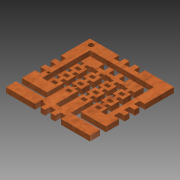
# Autodesk Inventor part: mech
Saved by Autodesk Inventor 2014 SP1 (Build 180222100, 222)
## iProperties
Created: 2015-02-17
Part Number: mech
Material: Wood (Cherry)
Document SubType Name: Modeling
Designer: Erin
Density: 0.63 g/cm^3
Appearance: Cherry - Natural Low Gloss
Author: Erin
Autodesk Inventor part; units mm, degrees
ref_plane "YZ Plane" through (0, 0, 0) normal (1, 0, 0) x (0, 1, 0)
ref_plane "XZ Plane" through (0, 0, 0) normal (0, 1, 0) x (-1, 0, 0)
ref_plane "XY Plane" through (0, 0, 0) normal (0, 0, 1) x (1, 0, 0)
sketch "slots" plane through (0, 0, 0) normal (0, 0, 1) x (1, 0, 0)
  line L0 (61.2817, 31.2571) -> (64.5817, 31.2571)
  line L1 (64.5817, 31.2571) -> (64.5817, 28.1071)
  line L2 (64.5817, 28.1071) -> (61.2817, 28.1071)
  line L3 (61.2817, 28.1071) -> (61.2817, 31.2571)
  line L4 (68.9317, 33.8834) -> (68.9317, 26.9198) construction
  line L5 (67.2817, 31.2571) -> (70.5817, 31.2571)
  line L6 (70.5817, 31.2571) -> (70.5817, 28.1071)
  line L7 (70.5817, 28.1071) -> (67.2817, 28.1071)
  line L8 (67.2817, 28.1071) -> (67.2817, 31.2571)
  line L9 (73.2817, 31.2571) -> (76.5817, 31.2571)
  line L10 (76.5817, 31.2571) -> (76.5817, 28.1071)
  line L11 (76.5817, 28.1071) -> (73.2817, 28.1071)
  line L12 (73.2817, 28.1071) -> (73.2817, 31.2571)
  line L13 (68.9317, 28.1071) -> (68.9317, 27.1937) construction
  point P0 (68.8645, 30.3856)
  dimension "d2" = 3.3
  dimension "d3" = 3.15
  dimension "d99" = 2.7
  dimension "d100" = 2.7
  measures "d2" distance of L1.end L2.end
  measures "d3" distance of L0.end L1.end
  measures "d99" distance between parallel lines of L8 L1
  measures "d100" distance between parallel lines of L12 L6
sketch "flexure" plane through (0, 0, 0) normal (0, 0, 1) x (1, 0, 0)
  line L0 (49.9032, 40.0133) -> (55.9032, 40.0133)
  line L1 (55.9032, 40.0133) -> (55.9032, 19.5133)
  line L2 (55.9032, 19.5133) -> (49.9032, 19.5133)
  line L3 (49.9032, 19.5133) -> (49.9032, 40.0133)
  line L4 (49.9032, 32.5133) -> (52.085, 32.5133)
  line L5 (52.085, 32.5133) -> (52.085, 30.5133)
  line L6 (52.085, 30.5133) -> (49.9032, 30.5133)
  line L7 (49.9032, 30.5133) -> (49.9032, 32.5133)
  line L8 (53.7214, 30.5133) -> (53.7214, 32.5133)
  line L9 (55.9032, 30.5133) -> (53.7214, 30.5133)
  line L10 (53.7214, 32.5133) -> (55.9032, 32.5133)
  line L11 (55.9032, 32.5133) -> (55.9032, 30.5133)
  line L12 (51.5395, 29.0133) -> (54.2668, 29.0133)
  line L13 (54.2668, 29.0133) -> (54.2668, 27.0133)
  line L14 (54.2668, 27.0133) -> (51.5395, 27.0133)
  line L15 (51.5395, 27.0133) -> (51.5395, 29.0133)
  line L16 (49.9032, 29.7633) -> (55.9032, 29.7633) construction
  line L17 (55.9032, 29.7633) -> (49.9032, 29.7633) construction
  line L18 (53.7214, 25.5133) -> (55.9032, 25.5133)
  line L19 (55.9032, 25.5133) -> (55.9032, 23.5133)
  line L20 (55.9032, 23.5133) -> (53.7214, 23.5133)
  line L21 (53.7214, 23.5133) -> (53.7214, 25.5133)
  line L22 (51.5395, 22.0133) -> (54.2668, 22.0133)
  line L23 (54.2668, 22.0133) -> (54.2668, 20.0133)
  line L24 (54.2668, 20.0133) -> (51.5395, 20.0133)
  line L25 (51.5395, 20.0133) -> (51.5395, 22.0133)
  line L26 (49.9032, 25.5133) -> (52.085, 25.5133)
  line L27 (52.085, 25.5133) -> (52.085, 23.5133)
  line L28 (52.085, 23.5133) -> (49.9032, 23.5133)
  line L29 (49.9032, 23.5133) -> (49.9032, 25.5133)
  line L30 (49.9032, 22.7633) -> (55.9032, 22.7633) construction
  line L31 (55.9032, 22.7633) -> (49.9032, 22.7633) construction
  line L32 (53.7214, 39.5133) -> (55.9032, 39.5133)
  line L33 (55.9032, 39.5133) -> (55.9032, 37.5133)
  line L34 (55.9032, 37.5133) -> (53.7214, 37.5133)
  line L35 (53.7214, 37.5133) -> (53.7214, 39.5133)
  line L36 (51.5395, 36.0133) -> (54.2668, 36.0133)
  line L37 (54.2668, 36.0133) -> (54.2668, 34.0133)
  line L38 (54.2668, 34.0133) -> (51.5395, 34.0133)
  line L39 (51.5395, 34.0133) -> (51.5395, 36.0133)
  line L40 (49.9032, 39.5133) -> (52.085, 39.5133)
  line L41 (52.085, 39.5133) -> (52.085, 37.5133)
  line L42 (52.085, 37.5133) -> (49.9032, 37.5133)
  line L43 (49.9032, 37.5133) -> (49.9032, 39.5133)
  line L44 (49.9032, 36.7633) -> (55.9032, 36.7633) construction
  line L45 (55.9032, 36.7633) -> (49.9032, 36.7633) construction
  line L46 (53.7214, 32.5133) -> (55.9032, 32.5133)
  line L47 (55.9032, 32.5133) -> (55.9032, 30.5133)
  line L48 (55.9032, 30.5133) -> (53.7214, 30.5133)
  line L49 (53.7214, 30.5133) -> (53.7214, 32.5133)
  line L50 (51.5395, 29.0133) -> (54.2668, 29.0133)
  line L51 (54.2668, 29.0133) -> (54.2668, 27.0133)
  line L52 (54.2668, 27.0133) -> (51.5395, 27.0133)
  line L53 (51.5395, 27.0133) -> (51.5395, 29.0133)
  line L54 (49.9032, 32.5133) -> (52.085, 32.5133)
  line L55 (52.085, 32.5133) -> (52.085, 30.5133)
  line L56 (52.085, 30.5133) -> (49.9032, 30.5133)
  line L57 (49.9032, 30.5133) -> (49.9032, 32.5133)
  line L58 (49.9032, 29.7633) -> (55.9032, 29.7633) construction
  line L59 (55.9032, 29.7633) -> (49.9032, 29.7633) construction
  point P0 (52.8239, 25.8216)
  dimension "d22" = 6
  dimension "d24" = 2.1818
  dimension "d27" = 3.8182
  dimension "d32" = 1.6364
  dimension "d33" = 2.7273
  dimension "d41" = 2
  dimension "d42" = 2
  dimension "d43" = 1.5
  dimension "d93" = 20.5
  dimension "d106" = 7
  dimension "d109" = 7
  dimension "d117" = 11
  measures "d22" distance of L1.end L2.end
  measures "d24" distance of L4.start L4.end
  measures "d27" distance of L6.end L9.end
  measures "d32" distance between parallel lines of L15 L3
  measures "d33" distance of L12.start L12.end
  measures "d41" distance of L4.end L5.end
  measures "d42" distance of L12.end L13.end
  measures "d43" distance between parallel lines of L12 L6
  measures "d93" distance of L0.end L1.end
  measures "d106" distance of L10.start L18.start
  measures "d109" distance of L10.start L32.start
  measures "d117" distance between parallel lines of L12 L0
sketch "Sketch1" plane through (0, 0, 0) normal (0, 0, 1) x (1, 0, 0)
  line L0 (-25, 25) -> (25, 25) construction
  line L1 (25, 25) -> (25, -25) construction
  line L2 (25, -25) -> (-25, -25) construction
  line L3 (-25, -25) -> (-25, 25) construction
  line L4 (-25, -25) -> (25, -25)
  line L5 (25, -25) -> (25, -19)
  line L6 (25, -19) -> (-25, -19)
  line L7 (-25, -19) -> (-25, -25)
  line L8 (0, 33.5916) -> (0, -39.9789) construction
  line L9 (-35.9054, 0) -> (42.6007, 0) construction
  line L10 (-25, 25) -> (25, 25)
  line L11 (25, 25) -> (25, 19)
  line L12 (25, 19) -> (-25, 19)
  line L13 (-25, 19) -> (-25, 25)
  line L14 (-25, 19) -> (-19, 19)
  line L15 (-19, 19) -> (-19, -15.5)
  line L16 (-19, -15.5) -> (-25, -15.5)
  line L17 (-25, -15.5) -> (-25, 19)
  line L18 (-19, -15.5) -> (-10, -15.5)
  line L19 (-10, -15.5) -> (-10, -9.5)
  line L20 (-10, -9.5) -> (-19, -9.5)
  line L21 (-19, -9.5) -> (-19, -15.5)
  line L22 (25, 19) -> (19, 19)
  line L23 (19, 19) -> (19, -15.5)
  line L24 (19, -15.5) -> (25, -15.5)
  line L25 (25, -15.5) -> (25, 19)
  line L26 (19, -15.5) -> (10, -15.5)
  line L27 (10, -15.5) -> (10, -9.5)
  line L28 (10, -9.5) -> (19, -9.5)
  line L29 (19, -9.5) -> (19, -15.5)
  line L30 (-16, 16) -> (16, 16)
  line L31 (16, 16) -> (16, 11)
  line L32 (16, 11) -> (-16, 11)
  line L33 (-16, 11) -> (-16, 16)
  line L34 (-7.5, -9.5) -> (-1.5, -9.5)
  line L35 (-1.5, -9.5) -> (-1.5, -19)
  line L36 (-1.5, -19) -> (-7.5, -19)
  line L37 (-7.5, -19) -> (-7.5, -9.5)
  line L38 (1.5, -9.5) -> (7.5, -9.5)
  line L39 (7.5, -9.5) -> (7.5, -19)
  line L40 (7.5, -19) -> (1.5, -19)
  line L41 (1.5, -19) -> (1.5, -9.5)
  line L42 (-68.1542, 16.5688) -> (-29.44, 16.5688) construction
  line L43 (-29.44, 16.5688) -> (-29.44, -5.0786) construction
  line L44 (-29.44, -5.0786) -> (-68.1542, -5.0786) construction
  line L45 (-68.1542, -5.0786) -> (-68.1542, 16.5688) construction
  circle A0 centre (-21.2866, 22) radius 1.5
  line L46 (-7.65, 25) -> (-4.35, 25)
  line L47 (-4.35, 25) -> (-4.35, 21.85)
  line L48 (-4.35, 21.85) -> (-7.65, 21.85)
  line L49 (-7.65, 21.85) -> (-7.65, 25)
  line L50 (0, 27.6263) -> (0, 20.6627) construction
  line L51 (-1.65, 25) -> (1.65, 25)
  line L52 (1.65, 25) -> (1.65, 21.85)
  line L53 (1.65, 21.85) -> (-1.65, 21.85)
  line L54 (-1.65, 21.85) -> (-1.65, 25)
  line L55 (4.35, 25) -> (7.65, 25)
  line L56 (7.65, 25) -> (7.65, 21.85)
  line L57 (7.65, 21.85) -> (4.35, 21.85)
  line L58 (4.35, 21.85) -> (4.35, 25)
  line L59 (0, 21.85) -> (0, 20.9366) construction
  line L60 (-7.65, -21.85) -> (-4.35, -21.85)
  line L61 (-4.35, -21.85) -> (-4.35, -25)
  line L62 (-4.35, -25) -> (-7.65, -25)
  line L63 (-7.65, -25) -> (-7.65, -21.85)
  line L64 (0, -19.2237) -> (0, -26.1873) construction
  line L65 (-1.65, -21.85) -> (1.65, -21.85)
  line L66 (1.65, -21.85) -> (1.65, -25)
  line L67 (1.65, -25) -> (-1.65, -25)
  line L68 (-1.65, -25) -> (-1.65, -21.85)
  line L69 (4.35, -21.85) -> (7.65, -21.85)
  line L70 (7.65, -21.85) -> (7.65, -25)
  line L71 (7.65, -25) -> (4.35, -25)
  line L72 (4.35, -25) -> (4.35, -21.85)
  line L73 (0, -25) -> (0, -25.9134) construction
  line L74 (-25, -7.65) -> (-25, -4.35)
  line L75 (-25, -4.35) -> (-21.85, -4.35)
  line L76 (-21.85, -4.35) -> (-21.85, -7.65)
  line L77 (-21.85, -7.65) -> (-25, -7.65)
  line L78 (-27.6263, 0) -> (-20.6627, 0) construction
  line L79 (-25, -1.65) -> (-25, 1.65)
  line L80 (-25, 1.65) -> (-21.85, 1.65)
  line L81 (-21.85, 1.65) -> (-21.85, -1.65)
  line L82 (-21.85, -1.65) -> (-25, -1.65)
  line L83 (-25, 4.35) -> (-25, 7.65)
  line L84 (-25, 7.65) -> (-21.85, 7.65)
  line L85 (-21.85, 7.65) -> (-21.85, 4.35)
  line L86 (-21.85, 4.35) -> (-25, 4.35)
  line L87 (-21.85, 0) -> (-20.9366, 0) construction
  line L88 (21.85, -7.65) -> (21.85, -4.35)
  line L89 (21.85, -4.35) -> (25, -4.35)
  line L90 (25, -4.35) -> (25, -7.65)
  line L91 (25, -7.65) -> (21.85, -7.65)
  line L92 (19.2237, 0) -> (26.1873, 0) construction
  line L93 (21.85, -1.65) -> (21.85, 1.65)
  line L94 (21.85, 1.65) -> (25, 1.65)
  line L95 (25, 1.65) -> (25, -1.65)
  line L96 (25, -1.65) -> (21.85, -1.65)
  line L97 (21.85, 4.35) -> (21.85, 7.65)
  line L98 (21.85, 7.65) -> (25, 7.65)
  line L99 (25, 7.65) -> (25, 4.35)
  line L100 (25, 4.35) -> (21.85, 4.35)
  line L101 (25, 0) -> (25.9134, 0) construction
  line L102 (-16, 11) -> (-10, 11)
  line L103 (-10, 11) -> (-10, -9.5)
  line L104 (-10, -9.5) -> (-16, -9.5)
  line L105 (-16, -9.5) -> (-16, 11)
  line L106 (-16, 3.5) -> (-13.8182, 3.5)
  line L107 (-13.8182, 3.5) -> (-13.8182, 1.5)
  line L108 (-13.8182, 1.5) -> (-16, 1.5)
  line L109 (-16, 1.5) -> (-16, 3.5)
  line L110 (-12.1818, 1.5) -> (-12.1818, 3.5)
  line L111 (-10, 1.5) -> (-12.1818, 1.5)
  line L112 (-12.1818, 3.5) -> (-10, 3.5)
  line L113 (-10, 3.5) -> (-10, 1.5)
  line L114 (-14.3636, 0) -> (-11.6364, 0)
  line L115 (-11.6364, 0) -> (-11.6364, -2)
  line L116 (-11.6364, -2) -> (-14.3636, -2)
  line L117 (-14.3636, -2) -> (-14.3636, 0)
  line L118 (-16, 0.75) -> (-10, 0.75) construction
  line L119 (-10, 0.75) -> (-16, 0.75) construction
  line L120 (-12.1818, -3.5) -> (-10, -3.5)
  line L121 (-10, -3.5) -> (-10, -5.5)
  line L122 (-10, -5.5) -> (-12.1818, -5.5)
  line L123 (-12.1818, -5.5) -> (-12.1818, -3.5)
  line L124 (-14.3636, -7) -> (-11.6364, -7)
  line L125 (-11.6364, -7) -> (-11.6364, -9)
  line L126 (-11.6364, -9) -> (-14.3636, -9)
  line L127 (-14.3636, -9) -> (-14.3636, -7)
  line L128 (-16, -3.5) -> (-13.8182, -3.5)
  line L129 (-13.8182, -3.5) -> (-13.8182, -5.5)
  line L130 (-13.8182, -5.5) -> (-16, -5.5)
  line L131 (-16, -5.5) -> (-16, -3.5)
  line L132 (-16, -6.25) -> (-10, -6.25) construction
  line L133 (-10, -6.25) -> (-16, -6.25) construction
  line L134 (-12.1818, 10.5) -> (-10, 10.5)
  line L135 (-10, 10.5) -> (-10, 8.5)
  line L136 (-10, 8.5) -> (-12.1818, 8.5)
  line L137 (-12.1818, 8.5) -> (-12.1818, 10.5)
  line L138 (-14.3636, 7) -> (-11.6364, 7)
  line L139 (-11.6364, 7) -> (-11.6364, 5)
  line L140 (-11.6364, 5) -> (-14.3636, 5)
  line L141 (-14.3636, 5) -> (-14.3636, 7)
  line L142 (-16, 10.5) -> (-13.8182, 10.5)
  line L143 (-13.8182, 10.5) -> (-13.8182, 8.5)
  line L144 (-13.8182, 8.5) -> (-16, 8.5)
  line L145 (-16, 8.5) -> (-16, 10.5)
  line L146 (-16, 7.75) -> (-10, 7.75) construction
  line L147 (-10, 7.75) -> (-16, 7.75) construction
  line L148 (-12.1818, 3.5) -> (-10, 3.5)
  line L149 (-10, 3.5) -> (-10, 1.5)
  line L150 (-10, 1.5) -> (-12.1818, 1.5)
  line L151 (-12.1818, 1.5) -> (-12.1818, 3.5)
  line L152 (-14.3636, 0) -> (-11.6364, 0)
  line L153 (-11.6364, 0) -> (-11.6364, -2)
  line L154 (-11.6364, -2) -> (-14.3636, -2)
  line L155 (-14.3636, -2) -> (-14.3636, 0)
  line L156 (-16, 3.5) -> (-13.8182, 3.5)
  line L157 (-13.8182, 3.5) -> (-13.8182, 1.5)
  line L158 (-13.8182, 1.5) -> (-16, 1.5)
  line L159 (-16, 1.5) -> (-16, 3.5)
  line L160 (-16, 0.75) -> (-10, 0.75) construction
  line L161 (-10, 0.75) -> (-16, 0.75) construction
  line L162 (10, 11) -> (16, 11)
  line L163 (16, 11) -> (16, -9.5)
  line L164 (16, -9.5) -> (10, -9.5)
  line L165 (10, -9.5) -> (10, 11)
  line L166 (10, 3.5) -> (12.1818, 3.5)
  line L167 (12.1818, 3.5) -> (12.1818, 1.5)
  line L168 (12.1818, 1.5) -> (10, 1.5)
  line L169 (10, 1.5) -> (10, 3.5)
  line L170 (13.8182, 1.5) -> (13.8182, 3.5)
  line L171 (16, 1.5) -> (13.8182, 1.5)
  line L172 (13.8182, 3.5) -> (16, 3.5)
  line L173 (16, 3.5) -> (16, 1.5)
  line L174 (11.6364, 0) -> (14.3636, 0)
  line L175 (14.3636, 0) -> (14.3636, -2)
  line L176 (14.3636, -2) -> (11.6364, -2)
  line L177 (11.6364, -2) -> (11.6364, 0)
  line L178 (10, 0.75) -> (16, 0.75) construction
  line L179 (16, 0.75) -> (10, 0.75) construction
  line L180 (13.8182, -3.5) -> (16, -3.5)
  line L181 (16, -3.5) -> (16, -5.5)
  line L182 (16, -5.5) -> (13.8182, -5.5)
  line L183 (13.8182, -5.5) -> (13.8182, -3.5)
  line L184 (11.6364, -7) -> (14.3636, -7)
  line L185 (14.3636, -7) -> (14.3636, -9)
  line L186 (14.3636, -9) -> (11.6364, -9)
  line L187 (11.6364, -9) -> (11.6364, -7)
  line L188 (10, -3.5) -> (12.1818, -3.5)
  line L189 (12.1818, -3.5) -> (12.1818, -5.5)
  line L190 (12.1818, -5.5) -> (10, -5.5)
  line L191 (10, -5.5) -> (10, -3.5)
  line L192 (10, -6.25) -> (16, -6.25) construction
  line L193 (16, -6.25) -> (10, -6.25) construction
  line L194 (13.8182, 10.5) -> (16, 10.5)
  line L195 (16, 10.5) -> (16, 8.5)
  line L196 (16, 8.5) -> (13.8182, 8.5)
  line L197 (13.8182, 8.5) -> (13.8182, 10.5)
  line L198 (11.6364, 7) -> (14.3636, 7)
  line L199 (14.3636, 7) -> (14.3636, 5)
  line L200 (14.3636, 5) -> (11.6364, 5)
  line L201 (11.6364, 5) -> (11.6364, 7)
  line L202 (10, 10.5) -> (12.1818, 10.5)
  line L203 (12.1818, 10.5) -> (12.1818, 8.5)
  line L204 (12.1818, 8.5) -> (10, 8.5)
  line L205 (10, 8.5) -> (10, 10.5)
  line L206 (10, 7.75) -> (16, 7.75) construction
  line L207 (16, 7.75) -> (10, 7.75) construction
  line L208 (13.8182, 3.5) -> (16, 3.5)
  line L209 (16, 3.5) -> (16, 1.5)
  line L210 (16, 1.5) -> (13.8182, 1.5)
  line L211 (13.8182, 1.5) -> (13.8182, 3.5)
  line L212 (11.6364, 0) -> (14.3636, 0)
  line L213 (14.3636, 0) -> (14.3636, -2)
  line L214 (14.3636, -2) -> (11.6364, -2)
  line L215 (11.6364, -2) -> (11.6364, 0)
  line L216 (10, 3.5) -> (12.1818, 3.5)
  line L217 (12.1818, 3.5) -> (12.1818, 1.5)
  line L218 (12.1818, 1.5) -> (10, 1.5)
  line L219 (10, 1.5) -> (10, 3.5)
  line L220 (10, 0.75) -> (16, 0.75) construction
  line L221 (16, 0.75) -> (10, 0.75) construction
  line L222 (1.5, 11) -> (7.5, 11)
  line L223 (7.5, 11) -> (7.5, -9.5)
  line L224 (7.5, -9.5) -> (1.5, -9.5)
  line L225 (1.5, -9.5) -> (1.5, 11)
  line L226 (1.5, 3.5) -> (3.6818, 3.5)
  line L227 (3.6818, 3.5) -> (3.6818, 1.5)
  line L228 (3.6818, 1.5) -> (1.5, 1.5)
  line L229 (1.5, 1.5) -> (1.5, 3.5)
  line L230 (5.3182, 1.5) -> (5.3182, 3.5)
  line L231 (7.5, 1.5) -> (5.3182, 1.5)
  line L232 (5.3182, 3.5) -> (7.5, 3.5)
  line L233 (7.5, 3.5) -> (7.5, 1.5)
  line L234 (3.1364, 0) -> (5.8636, 0)
  line L235 (5.8636, 0) -> (5.8636, -2)
  line L236 (5.8636, -2) -> (3.1364, -2)
  line L237 (3.1364, -2) -> (3.1364, 0)
  line L238 (1.5, 0.75) -> (7.5, 0.75) construction
  line L239 (7.5, 0.75) -> (1.5, 0.75) construction
  line L240 (5.3182, -3.5) -> (7.5, -3.5)
  line L241 (7.5, -3.5) -> (7.5, -5.5)
  line L242 (7.5, -5.5) -> (5.3182, -5.5)
  line L243 (5.3182, -5.5) -> (5.3182, -3.5)
  line L244 (3.1364, -7) -> (5.8636, -7)
  line L245 (5.8636, -7) -> (5.8636, -9)
  line L246 (5.8636, -9) -> (3.1364, -9)
  line L247 (3.1364, -9) -> (3.1364, -7)
  line L248 (1.5, -3.5) -> (3.6818, -3.5)
  line L249 (3.6818, -3.5) -> (3.6818, -5.5)
  line L250 (3.6818, -5.5) -> (1.5, -5.5)
  line L251 (1.5, -5.5) -> (1.5, -3.5)
  line L252 (1.5, -6.25) -> (7.5, -6.25) construction
  line L253 (7.5, -6.25) -> (1.5, -6.25) construction
  line L254 (5.3182, 10.5) -> (7.5, 10.5)
  line L255 (7.5, 10.5) -> (7.5, 8.5)
  line L256 (7.5, 8.5) -> (5.3182, 8.5)
  line L257 (5.3182, 8.5) -> (5.3182, 10.5)
  line L258 (3.1364, 7) -> (5.8636, 7)
  line L259 (5.8636, 7) -> (5.8636, 5)
  line L260 (5.8636, 5) -> (3.1364, 5)
  line L261 (3.1364, 5) -> (3.1364, 7)
  line L262 (1.5, 10.5) -> (3.6818, 10.5)
  line L263 (3.6818, 10.5) -> (3.6818, 8.5)
  line L264 (3.6818, 8.5) -> (1.5, 8.5)
  line L265 (1.5, 8.5) -> (1.5, 10.5)
  line L266 (1.5, 7.75) -> (7.5, 7.75) construction
  line L267 (7.5, 7.75) -> (1.5, 7.75) construction
  line L268 (5.3182, 3.5) -> (7.5, 3.5)
  line L269 (7.5, 3.5) -> (7.5, 1.5)
  line L270 (7.5, 1.5) -> (5.3182, 1.5)
  line L271 (5.3182, 1.5) -> (5.3182, 3.5)
  line L272 (3.1364, 0) -> (5.8636, 0)
  line L273 (5.8636, 0) -> (5.8636, -2)
  line L274 (5.8636, -2) -> (3.1364, -2)
  line L275 (3.1364, -2) -> (3.1364, 0)
  line L276 (1.5, 3.5) -> (3.6818, 3.5)
  line L277 (3.6818, 3.5) -> (3.6818, 1.5)
  line L278 (3.6818, 1.5) -> (1.5, 1.5)
  line L279 (1.5, 1.5) -> (1.5, 3.5)
  line L280 (1.5, 0.75) -> (7.5, 0.75) construction
  line L281 (7.5, 0.75) -> (1.5, 0.75) construction
  line L282 (-7.5, 11) -> (-1.5, 11)
  line L283 (-1.5, 11) -> (-1.5, -9.5)
  line L284 (-1.5, -9.5) -> (-7.5, -9.5)
  line L285 (-7.5, -9.5) -> (-7.5, 11)
  line L286 (-7.5, 3.5) -> (-5.3182, 3.5)
  line L287 (-5.3182, 3.5) -> (-5.3182, 1.5)
  line L288 (-5.3182, 1.5) -> (-7.5, 1.5)
  line L289 (-7.5, 1.5) -> (-7.5, 3.5)
  line L290 (-3.6818, 1.5) -> (-3.6818, 3.5)
  line L291 (-1.5, 1.5) -> (-3.6818, 1.5)
  line L292 (-3.6818, 3.5) -> (-1.5, 3.5)
  line L293 (-1.5, 3.5) -> (-1.5, 1.5)
  line L294 (-5.8636, 0) -> (-3.1364, 0)
  line L295 (-3.1364, 0) -> (-3.1364, -2)
  line L296 (-3.1364, -2) -> (-5.8636, -2)
  line L297 (-5.8636, -2) -> (-5.8636, 0)
  line L298 (-7.5, 0.75) -> (-1.5, 0.75) construction
  line L299 (-1.5, 0.75) -> (-7.5, 0.75) construction
  line L300 (-3.6818, -3.5) -> (-1.5, -3.5)
  line L301 (-1.5, -3.5) -> (-1.5, -5.5)
  line L302 (-1.5, -5.5) -> (-3.6818, -5.5)
  line L303 (-3.6818, -5.5) -> (-3.6818, -3.5)
  line L304 (-5.8636, -7) -> (-3.1364, -7)
  line L305 (-3.1364, -7) -> (-3.1364, -9)
  line L306 (-3.1364, -9) -> (-5.8636, -9)
  line L307 (-5.8636, -9) -> (-5.8636, -7)
  line L308 (-7.5, -3.5) -> (-5.3182, -3.5)
  line L309 (-5.3182, -3.5) -> (-5.3182, -5.5)
  line L310 (-5.3182, -5.5) -> (-7.5, -5.5)
  line L311 (-7.5, -5.5) -> (-7.5, -3.5)
  line L312 (-7.5, -6.25) -> (-1.5, -6.25) construction
  line L313 (-1.5, -6.25) -> (-7.5, -6.25) construction
  line L314 (-3.6818, 10.5) -> (-1.5, 10.5)
  line L315 (-1.5, 10.5) -> (-1.5, 8.5)
  line L316 (-1.5, 8.5) -> (-3.6818, 8.5)
  line L317 (-3.6818, 8.5) -> (-3.6818, 10.5)
  line L318 (-5.8636, 7) -> (-3.1364, 7)
  line L319 (-3.1364, 7) -> (-3.1364, 5)
  line L320 (-3.1364, 5) -> (-5.8636, 5)
  line L321 (-5.8636, 5) -> (-5.8636, 7)
  line L322 (-7.5, 10.5) -> (-5.3182, 10.5)
  line L323 (-5.3182, 10.5) -> (-5.3182, 8.5)
  line L324 (-5.3182, 8.5) -> (-7.5, 8.5)
  line L325 (-7.5, 8.5) -> (-7.5, 10.5)
  line L326 (-7.5, 7.75) -> (-1.5, 7.75) construction
  line L327 (-1.5, 7.75) -> (-7.5, 7.75) construction
  line L328 (-3.6818, 3.5) -> (-1.5, 3.5)
  line L329 (-1.5, 3.5) -> (-1.5, 1.5)
  line L330 (-1.5, 1.5) -> (-3.6818, 1.5)
  line L331 (-3.6818, 1.5) -> (-3.6818, 3.5)
  line L332 (-5.8636, 0) -> (-3.1364, 0)
  line L333 (-3.1364, 0) -> (-3.1364, -2)
  line L334 (-3.1364, -2) -> (-5.8636, -2)
  line L335 (-5.8636, -2) -> (-5.8636, 0)
  line L336 (-7.5, 3.5) -> (-5.3182, 3.5)
  line L337 (-5.3182, 3.5) -> (-5.3182, 1.5)
  line L338 (-5.3182, 1.5) -> (-7.5, 1.5)
  line L339 (-7.5, 1.5) -> (-7.5, 3.5)
  line L340 (-7.5, 0.75) -> (-1.5, 0.75) construction
  line L341 (-1.5, 0.75) -> (-7.5, 0.75) construction
  line L342 (-7.65, 16) -> (-4.35, 16)
  line L343 (-4.35, 16) -> (-4.35, 12.85)
  line L344 (-4.35, 12.85) -> (-7.65, 12.85)
  line L345 (-7.65, 12.85) -> (-7.65, 16)
  line L346 (0, 18.6263) -> (0, 11.6627) construction
  line L347 (-1.65, 16) -> (1.65, 16)
  line L348 (1.65, 16) -> (1.65, 12.85)
  line L349 (1.65, 12.85) -> (-1.65, 12.85)
  line L350 (-1.65, 12.85) -> (-1.65, 16)
  line L351 (4.35, 16) -> (7.65, 16)
  line L352 (7.65, 16) -> (7.65, 12.85)
  line L353 (7.65, 12.85) -> (4.35, 12.85)
  line L354 (4.35, 12.85) -> (4.35, 16)
  line L355 (0, 12.85) -> (0, 11.9366) construction
  point P0 (0, 0)
  point P1 (0, 25)
  point P2 (25, 0)
  point P3 (0, 16)
  point P4 (-4.5, -9.5)
  point P5 (-4.5, -9.5)
  point P6 (4.5, -9.5)
  point P7 (4.5, -9.5)
  dimension "d76" = 6
  dimension "d89" = 2.5
  dimension "d90" = 2.5
  dimension "d91" = 3
  dimension "d0" = 50
  dimension "d1" = 50
  dimension "d16" = 6
  dimension "d19" = 6
  dimension "d21" = 5
  dimension "d75" = 3
  dimension "d94" = 3
  dimension "d95" = 3.5
  dimension "d96" = 6
  dimension "d97" = 6
  dimension "d101" = 32
  dimension "d114" = 3
  constraints: 84 end point, 23 horizontal, 20 parallel, 11 perpendicular, 10 vertical, 5 equal length, 5 midpoint, 3 collinear, 2 coincident, 2 point on line, 2 vertical alignment, 1 centre point, 1 horizontal alignment, 4 other
  measures "d0" distance of L1.end L2.end
  measures "d1" distance of L0.end L1.end
  measures "d16" distance between parallel lines of L12 L10
  measures "d19" distance between parallel lines of L4 L6
  measures "d21" distance between parallel lines of L32 L30
  measures "d75" distance between parallel lines of L33 L15
  measures "d94" distance between parallel lines of L30 L12
  measures "d95" distance between parallel lines of L6 L16
  measures "d96" distance of L35.end L36.end
  measures "d97" distance of L39.end L40.end
  measures "d101" distance of L30.start L30.end
  measures "d114" diameter of A0
extrude "Extrusion4" add sketch "Sketch1" along normal blind 3 contours L7 L6 L5 L4 L70 L69 L72 L66 L65 L68 L61 L60 L63 | L37 L34 L35 L6 | L285 L310 L309 L308 L288 L287 L286 L324 L323 L322 L32 L283 L314 L317 L316 L292 L290 L291 L300 L303 L302 L34 | L41 L38 L39 L6 | L225 L250 L249 L248 L228 L227 L226 L264 L263 L262 L32 L223 L254 L257 L256 L232 L230 L231 L240 L243 L242 L38 | L32 L33 L30 L345 L344 L343 L350 L349 L348 L354 L353 L352 L31 | L103 L134 L137 L136 L112 L110 L111 L120 L123 L122 L20 L105 L130 L129 L128 L108 L107 L106 L144 L143 L142 L32 | L32 L163 L194 L197 L196 L172 L170 L171 L180 L183 L182 L28 L165 L190 L189 L188 L168 L167 L166 L204 L203 L202 | L19 L18 L15 L20 | L15 L16 L17 L77 L76 L75 L82 L81 L80 L86 L85 L84 L12 | L28 L23 L26 L27 | L12 L13 L10 L49 L48 L47 L54 L53 L52 L58 L57 L56 L11 | L12 L25 L98 L97 L100 L94 L93 L96 L89 L88 L91 L24 L23
equation "\"d2\" = mat - kerf"
equation "\"d3\" = mat - 0.5 * kerf"
equation "\"d22\" = flex_w"
equation "\"d24\" = 0.363636 * flex_w"
equation "\"d27\" = 0.636364 * flex_w"
equation "\"d32\" = 0.272727 * flex_w"
equation "\"d33\" = 0.454545 * flex_w"
equation "\"d41\" = line_w"
equation "\"d42\" = line_w"
equation "\"d43\" = line_sp"
equation "\"d93\" = flex_h"
equation "\"d89\" = flex_sp"
equation "\"d90\" = flex_sp"
equation "\"d16\" = structure_w"
equation "\"d19\" = structure_w"
equation "\"structure_w\" = 6"
equation "\"structure_sp\" = 8"
equation "\"flex_w\" = 6"
equation "\"flex_h\" = 20.5"
equation "\"line_w\" = 2"
equation "\"line_sp\" = 1.5"
equation "\"flex_sp\" = 2.5"
equation "\"mat\" = 3"
equation "\"kerf\" = -0.3"
body "Solid4"
